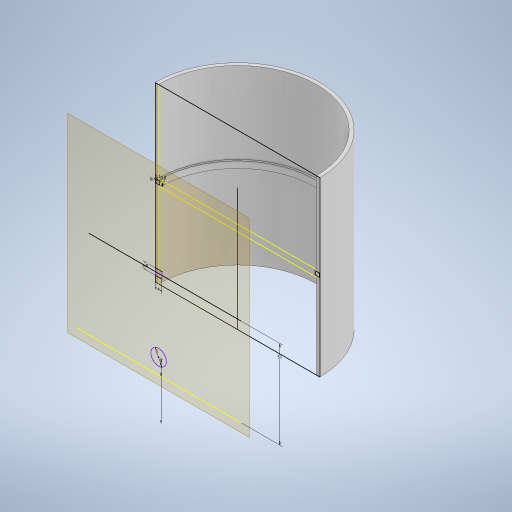
# Autodesk Inventor part: 탄두옆면1_2
Saved by Autodesk Inventor 2023 (Build 270158000, 158)
## iProperties
Created: 2023-10-31
Part Number: 탄두옆면1_2
Material: 일반
Document SubType Name: Modeling
Designer: rlatk
Density: 1 g/cm^3
Appearance: 기본값
Author: rlatk
Autodesk Inventor part; units mm, degrees
ref_plane "YZ Plane" through (0, 0, 0) normal (1, 0, 0) x (0, 1, 0)
ref_plane "XZ Plane" through (0, 0, 0) normal (0, 1, 0) x (-1, 0, 0)
sketch "스케치1" plane through (0, 0, 0) normal (0, 1, 0) x (-1, 0, 0)
  circle A0 centre (0, 0) radius 45.75
  circle A1 centre (0, 0) radius 47.75
  dimension "d0" = 91.5
  dimension "d1" = 2
  constraints: 2 centre point, 1 coincident
  measures "d0" diameter of A0
  measures "d1" radial gap between concentric circles of A0 A1
extrude "돌출1" add sketch "스케치1" along normal blind 100
ref_plane "작업 평면1" through (0, 0, 45.75) normal (0, 0, 1) x (1, 0, 0)
sketch "스케치2" plane through (0, 0, 45.75) normal (0, 0, 1) x (1, 0, 0)
  circle A0 centre (0, 9) radius 4.5
  line L0 (47.75, 0) -> (-47.75, 0) projected
  line L1 (-40.336, 51) -> (47.75, 51)
  line L2 (2, 52.9) -> (-2, 52.9)
  line L3 (-2, 52.9) -> (-2, 49.1)
  line L4 (-2, 49.1) -> (2, 49.1)
  line L5 (2, 49.1) -> (2, 52.9)
  line L6 (2, 52.9) -> (-2, 49.1) construction
  line L7 (-2, 52.9) -> (2, 49.1) construction
  point P0 (0, 0)
  point P1 (0, 51)
  dimension "d5" = 9
  dimension "d6" = 9
  dimension "d10" = 51
  dimension "d11" = 4
  dimension "d12" = 3.8
  constraints: 14 end point, 2 horizontal, 2 midpoint, 2 parallel, 1 centre point, 1 perpendicular, 1 point on line
  measures "d5" diameter of A0
  measures "d6" distance from line of L0 A0.centre
  measures "d10" distance between parallel lines of L1 L0
  measures "d11" distance of L4.end L3.end
  measures "d12" distance of L3.end L2.end
extrude "돌출2" add sketch "스케치2" against normal blind 10 contours A0
fillet "모깎기1" radius 2 1 edges at (-4.5, 9, 35.75)
sketch "스케치3" plane through (0, 0, 0) normal (1, 0, 0) x (0, 1, 0)
  line L0 (100, 45.75) -> (0, 45.75) projected
  line L1 (49.1, 45.75) -> (52.9, 45.75)
  line L2 (52.9, 45.75) -> (52.9, 44.75)
  line L3 (52.9, 44.75) -> (49.1, 44.75)
  line L4 (49.1, 44.75) -> (49.1, 45.75)
  line L5 (-20, 0) -> (120, 0) projected
  point P0 (0, 0)
  dimension "d15" = 1
  constraints: 8 end point, 2 parallel, 1 horizontal, 1 perpendicular
  measures "d15" distance of L1.end L2.end
revolve "회전1" add sketch "스케치3" angle 360 about axis through (0, -10, 0) along (0, 1, 0)
sketch "스케치4" plane through (0, 0, 0) normal (0, 0, 1) x (1, 0, 0)
  line L0 (47.75, 100) -> (-47.75, 100) projected
  line L1 (47.75, 0) -> (-47.75, 0) projected
  line L2 (-47.75, 100) -> (47.75, 100)
  line L3 (47.75, 100) -> (47.75, 0)
  line L4 (47.75, 0) -> (-47.75, 0)
  line L5 (-47.75, 0) -> (-47.75, 100)
  line L6 (-47.75, 0) -> (-47.75, 100) projected
  line L7 (-45.75, 49.1) -> (-45.75, 0) projected
  line L8 (-45.75, 100) -> (-45.75, 52.9) projected
  line L9 (-44.75, 52.9) -> (-44.75, 49.1) projected
  line L10 (45.75, 49.1) -> (-45.75, 49.1) projected
  line L11 (-45.75, 52.9) -> (45.75, 52.9) projected
  line L12 (-47.3, 49.9) -> (-45.2, 49.9)
  line L13 (-45.2, 49.9) -> (-45.2, 52)
  line L14 (-45.2, 52) -> (-47.3, 52)
  line L15 (-47.3, 52) -> (-47.3, 49.9)
  line L16 (0, 0) -> (0, 71.1344)
  line L17 (47.3, 49.9) -> (45.2, 49.9)
  line L18 (45.2, 49.9) -> (45.2, 52)
  line L19 (45.2, 52) -> (47.3, 52)
  line L20 (47.3, 52) -> (47.3, 49.9)
  dimension "d19" = 2.1
  dimension "d20" = 2.1
  dimension "d21" = 0.9
  dimension "d22" = 0.45
  constraints: 26 end point, 4 parallel, 4 symmetric about line, 2 horizontal, 2 perpendicular, 1 vertical
  measures "d19" distance of L14.end L13.end
  measures "d20" distance of L13.end L12.end
  measures "d21" distance between parallel lines of L11 L14
  measures "d22" distance between parallel lines of L15 L6
extrude "돌출4" cut sketch "스케치4" along normal blind 50 contours L3 L1 L16 L11 L8 L0 | L8 L11 L9 L10 L7 L1 L5 L0 | L1 L7 L10 L16 | L11 L16 L10 L9 | L15 L14 L13 L12 | L17 L18 L19 L20
extrude "돌출5" cut sketch "스케치4" against normal blind 2.1 contours L15 L14 L13 L12 | L17 L18 L19 L20
